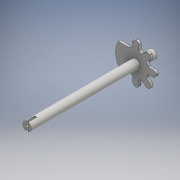
# Autodesk Inventor part: Main turning shaft
Saved by Autodesk Inventor 2016 (Build 200138000, 138)
## iProperties
Created: 2016-11-05
Part Number: Main turning shaft
Material: Generic
Document SubType Name: Modeling
Designer: Muhammad
Density: 1 g/cm^3
Appearance: Chrome - Polished
Author: Muhammad
Autodesk Inventor part; units mm, degrees
ref_plane "YZ Plane" through (0, 0, 0) normal (1, 0, 0) x (0, 1, 0)
ref_plane "XZ Plane" through (0, 0, 0) normal (0, 1, 0) x (-1, 0, 0)
ref_plane "XY Plane" through (0, 0, 0) normal (0, 0, 1) x (1, 0, 0)
sketch "Sketch1" plane through (0, 0, 0) normal (0, 1, 0) x (-1, 0, 0)
  point P0 (0, 0)
sketch "Sketch2" plane through (0, 0, 0) normal (0, 1, 0) x (-1, 0, 0)
  circle A0 centre (0, 0) radius 2
  dimension "d0" = 4
  constraints: 1 centre point, 1 coincident
  measures "d0" diameter of A0
extrude "Extrusion1" add sketch "Sketch2" along normal blind 51
sketch "Sketch3" plane through (0, 0, 0) normal (0, -1, 0) x (1, 0, 0)
  line L0 (-0.5, 2) -> (0.5, 2)
  line L1 (0.5, 2) -> (0.5, -2)
  line L2 (0.5, -2) -> (-0.5, -2)
  line L3 (-0.5, -2) -> (-0.5, 2)
  line L4 (-0.5, 2) -> (0.5, -2) construction
  line L5 (0.5, 2) -> (-0.5, -2) construction
  point P0 (0, 0)
  dimension "d3" = 1
  dimension "d4" = 4
  constraints: 12 end point, 2 midpoint, 2 parallel, 1 horizontal, 1 perpendicular
  measures "d3" distance of L1.end L2.end
  measures "d4" distance of L0.end L1.end
extrude "Extrusion2" cut sketch "Sketch3" against normal blind 4
sketch "Sketch4" plane through (0, 51, 0) normal (0, 1, 0) x (1, 0, 0)
  line L0 (0, 9.5) -> (0, -9.5) construction
  line L1 (9.5, 0) -> (-9.5, 0) construction
  line L2 (9.5, 0) -> (9.3816, 1.4953)
  line L3 (9.3816, 1.4953) -> (5.8107, 1.4953)
  line L4 (9.5, 0) -> (9.3816, -1.4953)
  line L5 (9.3816, -1.4953) -> (5.8107, -1.4953)
  line L6 (1.4882, -5.8125) -> (1.4882, -9.3827)
  line L7 (-1.4882, -5.8125) -> (-1.4882, -9.3827)
  line L8 (1.4882, 5.8125) -> (1.4882, 9.3827)
  line L9 (-1.4882, 5.8125) -> (-1.4882, 9.3827)
  line L10 (7.659, -5.6204) -> (4.9964, -3.322)
  line L11 (7.659, -5.6204) -> (6.6789, -6.7559)
  line L12 (6.6789, -6.7559) -> (5.5323, -7.723)
  line L13 (5.5323, -7.723) -> (2.7851, -5.3144)
  line L14 (7.659, 5.6204) -> (4.9964, 3.322)
  line L15 (5.5323, 7.723) -> (2.7851, 5.3144)
  line L16 (-9.5, 0) -> (-9.5, 5) construction
  line L17 (-9.5, 0) -> (-9.5, -5) construction
  line L18 (-8.0777, 5) -> (-3.0777, 5)
  line L19 (-8.0777, -5) -> (-3.0777, -5)
  line L20 (-1.4882, 5.8125) -> (-3.0777, 5)
  line L21 (-3.0777, -5) -> (-1.4882, -5.8125)
  arc A0 (-8.0777, 5) -> (-8.0777, -5) centre (0, 0) ccw
  arc A1 (-1.4882, -9.3827) -> (1.4882, -9.3827) centre (0, 0) ccw
  arc A2 (5.5323, -7.723) -> (7.659, -5.6204) centre (0, 0) ccw
  arc A3 (9.3816, -1.4953) -> (9.3816, 1.4953) centre (0, 0) ccw
  arc A4 (7.659, 5.6204) -> (5.5323, 7.723) centre (0, 0) ccw
  arc A5 (1.4882, 9.3827) -> (-1.4882, 9.3827) centre (0, 0) ccw
  arc A6 (5.8107, 1.4953) -> (4.9964, 3.322) centre (0, 0) ccw
  arc A7 (4.9964, -3.322) -> (5.8107, -1.4953) centre (0, 0) ccw
  arc A8 (1.4882, -5.8125) -> (2.7851, -5.3144) centre (0, 0) ccw
  arc A9 (2.7851, 5.3144) -> (1.4882, 5.8125) centre (0, 0) ccw
  dimension "d28" = 5
  dimension "d29" = 5
  constraints: 44 end point, 25 point on circle, 10 centre point, 8 symmetric about line, 4 horizontal, 2 coincident, 2 parallel, 2 vertical, 1 perpendicular, 1 tangent
  measures "d28" distance of L18.start L18.end
  measures "d29" distance of L19.start L19.end
extrude "Extrusion3" add sketch "Sketch4" along normal blind 1 contours L4 L5 A7 L10 L11 L12 L13 A8 L6 A1 L7 L21 L19 A0 L18 L20 L9 A5 L8 A9 L15 A4 L14 A6 L3 L2
fillet "Fillet1" radius 1.4 10 edges at (1.4882, 51.5, 9.3827) (-1.4882, 51.5, 9.3827) (9.3816, 51.5, 1.4953) (9.3816, 51.5, -1.4953) (7.659, 51.5, -5.6204) (5.5323, 51.5, -7.723) (1.4882, 51.5, -9.3827) (-1.4882, 51.5, -9.3827) (5.5323, 51.5, 7.723) (7.659, 51.5, 5.6204)
sketch "Sketch5" plane through (0, 52, 0) normal (0, 1, 0) x (1, 0, 0)
  circle A0 centre (0, 0) radius 2
  dimension "d33" = 4
  constraints: 1 centre point, 1 coincident
  measures "d33" diameter of A0
extrude "Extrusion4" add sketch "Sketch5" along normal blind 7
body "Solid1"
